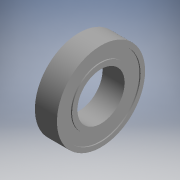
# Autodesk Inventor part: C6902ZZ
Saved by Autodesk Inventor 2017.3 (Build 213256000, 256)
## iProperties
Part Number: C6902ZZ
Material: Generic
Catalog Web Link: www.cadenas.de
Description: C6900ZZ,C6000ZZ,C6200ZZ,C6300ZZ,C6901ZZ,C6001ZZ,C6201ZZ,C6301ZZ,C6902ZZ,C6002ZZ,C6202ZZ,C6302ZZ,C6903ZZ,C6003ZZ,C6203ZZ,C6303ZZ,C6904ZZ,C6004ZZ,C6204ZZ,C6304ZZ,C6905ZZ,C6005ZZ,C6205ZZ,C6305ZZ,C6906ZZ,C6006ZZ,C6206ZZ,C6306ZZ-Deep Groove Ball Bearings (Economy) -Double Shielded-
Vendor: MISUMI
Document SubType Name: Modeling
Designer: partserver
Manufacturer: MISUMI
Mass: 2.92219 g
Surface Area: 19.1389 cm^2
Volume: 2.92219 cm^3
Density: 1 g/cm^3
Appearance: PSOLRGB-192-192-192
Category: PARTsolutions
Company: MISUMI
Title: C6902ZZ
Author: Cadenas PARTsolutions
Comments: Deep Groove Ball Bearings (Economy) -Double Shielded-
PSOL_IDENT_0: {$CADENAS_DATA\23d-libs\misumi\metric\12_bearing_holders\c6900zz.prj},371 {VTYP=3D},{NB=C6902ZZ},{LI
PSOL_IDENT_1: NA=C6902ZZ},{NN=C6900ZZ,C6000ZZ,C6200ZZ,C6300ZZ,C6901ZZ,C6001ZZ,C6201ZZ,C6301ZZ,C6902ZZ,C6002ZZ,C620
PSOL_IDENT_2: 2ZZ,C6302ZZ,C6903ZZ,C6003ZZ,C6203ZZ,C6303ZZ,C6904ZZ,C6004ZZ,C6204ZZ,C6304ZZ,C6905ZZ,C6005ZZ,C6205ZZ,
PSOL_IDENT_3: C6305ZZ,C6906ZZ,C6006ZZ,C6206ZZ,C6306ZZ},{DATE=30.06.2021 12:58:26},{GEOMDATE=04.10.2012 04:14:00},{
PSOL_IDENT_4: VERSION=},{LINEID=90},{WBVAR=},{WBNUMERIC=}  {NB=C6902ZZ},{LINA=C6902ZZ},{KT=DUMMY},{PN=C6902ZZ},{BN=
PSOL_IDENT_5: 6902},{DD=15},{D=28},{B=7},{RR=0.3},{DEEP=0.330},{T1=3.350},{T2=9.200}
NB: C6902ZZ
NN: C6900ZZ,C6000ZZ,C6200ZZ,C6300ZZ,C6901ZZ,C6001ZZ,C6201ZZ,C6301ZZ,C6902ZZ,C6002ZZ,C6202ZZ,C6302ZZ,C6903ZZ,C6003ZZ,C6203ZZ,C6303ZZ,C6904ZZ,C6004ZZ,C6204ZZ,C6304ZZ,C6905ZZ,C6005ZZ,C6205ZZ,C6305ZZ,C6906ZZ,C6006ZZ,C6206ZZ,C6306ZZ
NT: Deep Groove Ball Bearings (Economy) -Double Shielded-
NBSYN: $PN.
LINA: C6902ZZ
CATALOG: Misumi
PN: C6902ZZ
DD: 15
D: 28
B: 7
RR: 0.3
SUPPLIER: MISUMI
ARTICLENO: C6902ZZ
BOMINFO: C6902ZZ
CREATOR: CADENAS GmbH
Autodesk Inventor part; units mm, degrees
sketch "Sketch_1" plane through (0, 0, 0) normal (0, 0, 1) x (1, 0, 0)
  line L0 (50, 0) -> (-50, 0)
  line L1 (0, 12.55) -> (0.33, 12.55)
  line L2 (0.33, 12.55) -> (0.33, 9.2)
  line L3 (0.33, 9.2) -> (0, 9.2)
  line L4 (0, 9.2) -> (0, 7.5)
  line L5 (0, 7.5) -> (7, 7.5)
  line L6 (7, 7.5) -> (7, 9.2)
  line L7 (7, 9.2) -> (6.67, 9.2)
  line L8 (6.67, 9.2) -> (6.67, 12.55)
  line L9 (6.67, 12.55) -> (7, 12.55)
  line L10 (7, 12.55) -> (7, 14)
  line L11 (7, 14) -> (0, 14)
  line L12 (0, 14) -> (0, 12.55)
  constraints: 26 end point
revolve "Revolution1" add sketch "Sketch_1" angle 360 about axis through (50, 0, 0) along (1, 0, 0)
ref_plane "to_cp1_XY" through (0, 0, 0) normal (1, 0, 0) x (0, 0, -1)
ref_plane "to_cp1_YZ" through (0, 0, 0) normal (0, 0, -1) x (0, 1, 0)
ref_plane "to_cp1_ZX" through (0, 0, 0) normal (0, 1, 0) x (1, 0, 0)
body "Solid1"
